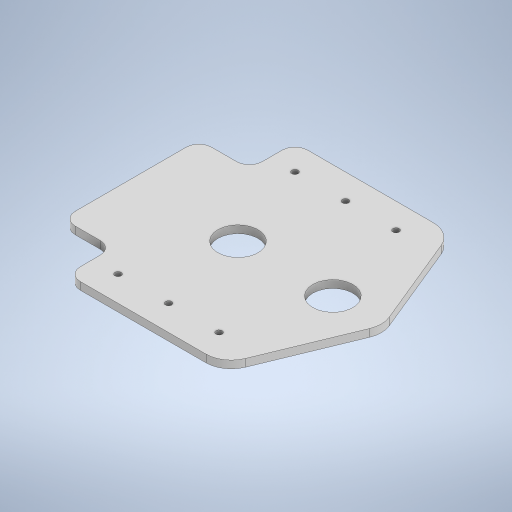
# Autodesk Inventor part: AntennaPlateUpper
Saved by Autodesk Inventor 2023 (Build 270158000, 158)
## iProperties
Created: 2022-11-29
Part Number: AntennaPlateUpper
Material: Generic
Document SubType Name: Modeling
Designer: Administrator
Density: 1 g/cm^3
Appearance: Default
Author: Administrator
Autodesk Inventor part; units mm, degrees
ref_plane "YZ Plane" through (0, 0, 0) normal (1, 0, 0) x (0, 1, 0)
ref_plane "XZ Plane" through (0, 0, 0) normal (0, 1, 0) x (-1, 0, 0)
ref_plane "XY Plane" through (0, 0, 0) normal (0, 0, 1) x (1, 0, 0)
sketch "Sketch1" plane through (0, 0, 0) normal (0, 1, 0) x (-1, 0, 0)
  line L0 (15.1833, 0) -> (65, 0)
  line L1 (90, 0) -> (90, -18) construction
  line L2 (90, -90) -> (70, -90) construction
  line L3 (0, -90) -> (0, 0) construction
  line L4 (85, -18) -> (75, -18)
  line L5 (70, -18) -> (70, -72) construction
  line L6 (75, -72) -> (85, -72)
  line L7 (90, -67) -> (90, -18)
  circle A0 centre (80, -10) radius 10 construction
  circle A1 centre (80, -80) radius 10 construction
  circle A2 centre (80, -10) radius 1.25
  circle A3 centre (80, -80) radius 1.25
  circle A4 centre (60, -10) radius 1.25
  circle A5 centre (60, -80) radius 1.25
  circle A6 centre (40, -10) radius 1.25
  circle A7 centre (40, -80) radius 1.25
  circle A8 centre (20, -10) radius 1.25
  circle A9 centre (20, -80) radius 1.25
  circle A10 centre (0, -10) radius 1.25 construction
  circle A11 centre (0, -80) radius 1.25 construction
  line L8 (20, -10) -> (0, -80) construction
  circle A12 centre (10, -45) radius 7.9375
  circle A13 centre (10, -45) radius 20 construction
  line L9 (0, 0) -> (-10, 0) construction
  line L10 (-10, 0) -> (-10, -90) construction
  line L11 (-10, -90) -> (0, -90) construction
  circle A14 centre (1, -9) radius 3.5 construction
  circle A15 centre (1, -81) radius 3.5 construction
  line L12 (4.5, -90) -> (4.5, -81) construction
  line L13 (4.5, 0) -> (4.5, -9) construction
  line L14 (-8.44, -48.7987) -> (4.2376, -79.6704)
  line L15 (-8.44, -41.2013) -> (4.2376, -10.3296)
  line L16 (4.2376, -10.3296) -> (5.9329, -6.2013)
  line L17 (4.2376, -79.6704) -> (5.9329, -83.7987)
  arc A16 (15.1833, 0) -> (5.9329, -6.2013) centre (15.1833, -10) ccw
  arc A17 (5.9329, -83.7987) -> (15.1833, -90) centre (15.1833, -80) ccw
  arc A18 (-8.44, -41.2013) -> (-8.44, -48.7987) centre (0.8104, -45) ccw
  line L18 (90, -23) -> (90, -72)
  line L19 (90, -72) -> (90, -90) construction
  line L20 (70, -13) -> (70, -5)
  line L21 (70, -77) -> (70, -85)
  line L22 (65, -90) -> (15.1833, -90)
  arc A19 (70, -5) -> (65, 0) centre (65, -5) ccw
  arc A20 (70, -13) -> (75, -18) centre (75, -13) ccw
  arc A21 (90, -23) -> (85, -18) centre (85, -23) ccw
  arc A22 (85, -72) -> (90, -67) centre (85, -67) ccw
  arc A23 (75, -72) -> (70, -77) centre (75, -77) ccw
  arc A24 (65, -90) -> (70, -85) centre (65, -85) ccw
  line L23 (10, -45) -> (47.545, -45) construction
  circle A25 centre (47.545, -45) radius 7.9375
  point P0 (-10, -45)
  point P1 (8.4795, 0)
  point P2 (8.4795, -90)
  dimension "d0" = 90
  dimension "d1" = 90
  dimension "d2" = 20
  dimension "d3" = 54
  dimension "d4" = 18
  dimension "d5" = 2.5
  dimension "d8" = 70
  dimension "d11" = 20
  dimension "d14" = 15.875
  dimension "d15" = 40
  dimension "d17" = 7
  dimension "d18" = 89
  dimension "d19" = 7
  dimension "d20" = 0
  dimension "d21" = 72
  dimension "d22" = 9
  dimension "d23" = 10
  dimension "d24" = 10
  dimension "d25" = 5
  dimension "d26" = 37.545
  dimension "d27" = 15.875
  constraints: 48 end point, 33 tangent, 26 centre point, 26 point on line, 22 point on circle, 7 parallel, 7 perpendicular, 6 equal radius, 5 horizontal, 3 coincident, 2 midpoint, 1 vertical, 18 other
  measures "d0" distance of L2.start L3.start
  measures "d1" distance of L1.start L2.start
  measures "d2" distance of L18.end L5.end
  measures "d3" distance of L5.end L5.start
  measures "d4" distance between parallel lines of L0 L4
  measures "d5" diameter of A2
  measures "d8" distance of A2.centre A3.centre
  measures "d11" distance of A2.centre A4.centre
  measures "d14" diameter of A12
  measures "d15" diameter of A13
  measures "d17" diameter of A14
  measures "d18" distance from line of L1 A14.centre
  measures "d19" diameter of A15
  measures "d20" horizontal distance of A15.centre A14.centre
  measures "d21" distance of A15.centre A14.centre
  measures "d22" distance from line of L2 A15.centre
  measures "d23" radius of A16
  measures "d24" radius of A18
  measures "d25" radius of A19
  measures "d26" distance of L23.start L23.end
  measures "d27" diameter of A25
extrude "Extrusion1" add sketch "Sketch1" along normal blind 3 contours L0 A19 L20 A20 L4 A21 L7 A22 L6 A23 L21 A24 L22 A17 L17 L14 A18 L15 L16 A16
equation "\"d4\" = -0.5 * d3 + 0.5 * d1"
equation "\"d22\" = -0.5 * d21 + 0.5 * d1"
equation "\"d27\" = d14"
body "Solid1"
